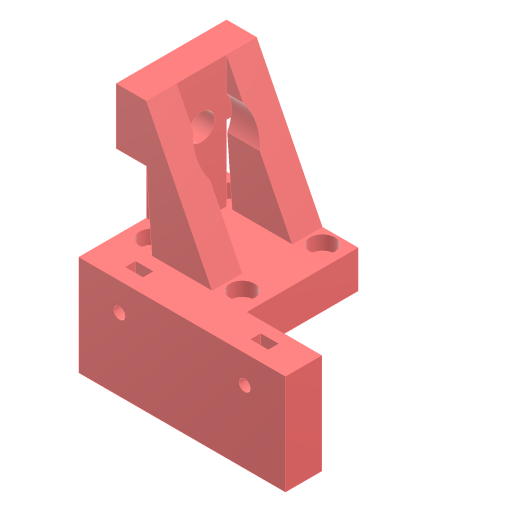
# Autodesk Inventor part: Part1
Saved by Autodesk Inventor 2024.3 (Build 283343000, 343)
## iProperties
Created: 2025-03-29
Part Number: Part1
Material: PC/ABS Plastic
Document SubType Name: Modeling
Designer: MPA
Density: 1.1 g/cm^3
Appearance: Smooth - Red
Mass: 105.816 g
Surface Area: 229.328 cm^2
Volume: 96.196 cm^3
Author: MPA
## iProperties of the stored document Part1_3DPrint.ipt
Created: 2025-06-18
Part Number: Part1_3DPrint
Material: Generic
Document SubType Name: Modeling
Designer: MPA
Density: 1 g/cm^3
Appearance: Default
Author: MPA
Autodesk Inventor part; units mm, degrees
ref_plane "YZ Plane" through (0, 0, 0) normal (1, 0, 0) x (0, 1, 0)
ref_plane "XZ Plane" through (0, 0, 0) normal (0, 1, 0) x (-1, 0, 0)
ref_plane "XY Plane" through (0, 0, 0) normal (0, 0, 1) x (1, 0, 0)
sketch "Sketch1" plane through (0, 0, 0) normal (0, 1, 0) x (-1, 0, 0)
  line L0 (-26.25, 22) -> (26.25, 22)
  line L1 (26.25, 22) -> (26.25, -22)
  line L2 (26.25, -22) -> (-26.25, -22)
  line L3 (-26.25, -22) -> (-26.25, 22)
  line L4 (-26.25, 22) -> (26.25, -22) construction
  line L5 (26.25, 22) -> (-26.25, -22) construction
  point P0 (0, 0)
  dimension "d0" = 44
  dimension "d1" = 52.5
  constraints: 12 end point, 2 midpoint, 2 parallel, 1 horizontal, 1 perpendicular
  measures "d0" distance of L0.end L1.end
  measures "d1" distance of L1.end L2.end
extrude "Extrusion1" add sketch "Sketch1" along normal blind 67.5
sketch "Sketch2" plane through (0, 67.5, 0) normal (0, 1, 0) x (1, 0, 0)
  line L0 (18, -16) -> (-18, -16) construction
  line L1 (-18, -16) -> (-18, 16) construction
  line L2 (-18, 16) -> (18, 16) construction
  line L3 (18, 16) -> (18, -16) construction
  line L4 (18, -16) -> (-18, 16) construction
  line L5 (-18, -16) -> (18, 16) construction
  point P0 (0, 0)
  point P1 (-18, 16)
  dimension "d4" = 32
  dimension "d5" = 36
  constraints: 12 end point, 4 coincident, 2 midpoint, 2 parallel, 1 horizontal, 1 perpendicular
  measures "d4" distance of L0.end L1.end
  measures "d5" distance of L1.end L2.end
hole "Hole1" at (-18, 67.5, -16) at (-18, 67.5, 16) at (18, 67.5, 16) at (18, 67.5, -16) direction (0, -1, 0) diameter 5.6 end through all
sketch "Sketch3" plane through (-26.25, 0, -22) normal (-1, 0, 0) x (0, 0, 1)
  line L0 (0, 0) -> (44, 0) projected
  line L1 (44, 0) -> (44, 67.5) projected
  line L2 (0, 67.5) -> (44, 67.5) projected
  line L3 (0, 0) -> (0, 67.5) projected
  point P0 (22, 0)
  point P1 (22, 47.5)
  point P2 (22, 0)
  dimension "d13" = 47.5
  constraints: 1 midpoint, 1 vertical alignment
  measures "d13" distance from line of L0 point (22, 47.5)
hole "Hole2" at (-26.25, 47.5, 0) direction (1, 0, 0) diameter 10.5 end through all
sketch "Sketch4" plane through (0, 67.5, 0) normal (0, 1, 0) x (1, 0, 0)
  circle A0 centre (18, 16) radius 2.8 projected
  circle A1 centre (18, -16) radius 2.8 projected
  circle A2 centre (-18, -16) radius 2.8 projected
  circle A3 centre (-18, 16) radius 2.8 projected
  line L0 (26.25, 22) -> (-26.25, 22) projected
  line L1 (-26.25, 22) -> (-26.25, -22) projected
  line L2 (-26.25, -22) -> (26.25, -22) projected
  line L3 (26.25, -22) -> (26.25, 22) projected
  line L4 (26.25, 22) -> (-14.25, 22)
  line L5 (-14.25, 22) -> (-14.25, -22)
  line L6 (-14.25, -22) -> (26.25, -22)
  line L7 (26.25, -22) -> (26.25, 22)
  line L8 (-26.25, 22) -> (-14.25, 22)
  line L9 (-14.25, 22) -> (-14.25, 10)
  line L10 (-14.25, 10) -> (-26.25, 10)
  line L11 (-26.25, 10) -> (-26.25, 22)
  line L12 (-14.25, -22) -> (-26.25, -22)
  line L13 (-26.25, -22) -> (-26.25, -10)
  line L14 (-26.25, -10) -> (-14.25, -10)
  line L15 (-14.25, -10) -> (-14.25, -22)
  point P0 (0, 0)
  dimension "d21" = 12
  dimension "d22" = 6
  dimension "d23" = 6
  dimension "d24" = 6
  constraints: 24 end point, 6 parallel, 3 horizontal, 3 perpendicular, 3 point on line
  measures "d21" distance between parallel lines of L1 L5
  measures "d22" distance from line of L0 A3.centre
  measures "d23" distance from line of L10 A3.centre
  measures "d24" distance from line of A2.centre L14
extrude "Extrusion2" cut sketch "Sketch4" against normal blind 52.5 contours L3 L2 L5 L0 | L5 L10 L1 L0 | L2 L1 L14 L5
sketch "Sketch5" plane through (-26.25, 67.5, 10) normal (0, 0, 1) x (1, 0, 0)
  line L0 (0, 0) -> (12, 0) projected
  line L1 (0, -52.5) -> (0, 0) projected
  line L2 (0, -52.5) -> (12, -52.5) projected
  line L3 (12, 0) -> (12, -52.5) projected
  line L4 (52.5, -52.5) -> (0, -52.5) projected
  line L5 (11.05, -52.5) -> (5.45, -52.5) projected
  line L6 (8.25, -52.5) -> (8.25, 0) construction
  line L7 (12, -22.5) -> (14.25, -52.5)
  line L8 (12, 0) -> (38.25, -52.5)
  line L9 (47.05, -52.5) -> (41.45, -52.5) projected
  line L10 (44.25, -52.5) -> (44.25, -22.1018) construction
  line L11 (12, -22.5) -> (0, -22.5)
  line L12 (0, -22.5) -> (0, 0)
  line L13 (0, 0) -> (12, 0)
  line L14 (38.25, -52.5) -> (14.25, -52.5)
  point P0 (26.25, -67.5)
  dimension "d27" = 30
  dimension "d28" = 36
  dimension "d29" = 6
  dimension "d30" = 6
  constraints: 16 end point, 5 point on line, 4 perpendicular, 2 midpoint, 1 collinear, 1 vertical
  measures "d27" distance from line of L4 L7.start
  measures "d28" distance between parallel lines of L10 L6
  measures "d29" distance from line of L10 L8.end
  measures "d30" distance from line of L6 L7.end
extrude "Extrusion3" add sketch "Sketch5" along normal up to surface (12 mm away) contours L0 L3 L11 L1 | L8 L4 L7 L3
sketch "Sketch6" plane through (0, 15, 0) normal (0, 1, 0) x (1, 0, 0)
  circle A0 centre (-18, -16) radius 2.8 projected
  circle A1 centre (18, -16) radius 2.8 projected
  circle A2 centre (18, 16) radius 2.8 projected
  circle A3 centre (-18, 16) radius 2.8 projected
  circle A4 centre (-18, 16) radius 2.8 projected
  point P0 (0, 0)
hole "Hole3" at (-18, 15, 16) at (18, 15, -16) at (-18, 15, -16) at (18, 15, 16) direction (0, -1, 0) diameter 5.5 end through all counterbore diameter 10 counterbore depth 5.7 clearance for "Socket Head Cap Screw ISO 4762" size "M5" standard "ISO"
mirror "Mirror1" about plane through (0, 0, 0) normal (0, 0, 1) of "Extrusion3"
sketch "Sketch7" plane through (-14.25, 15, 10) normal (1, 0, 0) x (0, 0, -1)
  circle A0 centre (10, 32.5) radius 5.25 projected
  circle A1 centre (10, 32.5) radius 12
  point P0 (10, -15)
  dimension "d40" = 24
  constraints: 1 centre point, 1 coincident
  measures "d40" diameter of A1
extrude "Extrusion4" cut sketch "Sketch7" along normal through all contours A0 | A1
sketch "Sketch8" plane through (-26.25, 0, 22) normal (0, 0, 1) x (1, 0, 0)
  line L0 (52.5, 15) -> (38.25, 15) projected
  line L1 (12, 67.5) -> (38.25, 15) projected
  line L2 (0, 67.5) -> (12, 67.5) projected
  line L3 (0, 45) -> (0, 67.5) projected
  line L4 (12, 45) -> (0, 45) projected
  line L5 (14.25, 15) -> (12, 45) projected
  line L6 (14.25, 15) -> (0, 15) projected
  line L7 (0, 0) -> (0, 15) projected
  line L8 (0, 0) -> (52.5, 0) projected
  line L9 (52.5, 0) -> (52.5, 15) projected
  line L10 (14.25, 15) -> (38.25, 15)
  point P0 (26.25, 0)
  constraints: 2 end point, 1 collinear
extrude "Extrusion5" add sketch "Sketch8" along normal blind 15 contours L9 L8 L7 L6 L10 L0
sketch "Sketch9" plane through (0, 0, 0) normal (0, -1, 0) x (1, 0, 0)
  circle A0 centre (18, -16) radius 2.8 projected
  circle A1 centre (18, 16) radius 2.8 projected
  circle A2 centre (-18, 16) radius 2.8 projected
  circle A3 centre (-18, -16) radius 2.8 projected
  line L0 (26.25, -22) -> (-26.25, -22) projected
  line L1 (26.25, -22) -> (26.25, 37) projected
  line L2 (-26.25, 37) -> (26.25, 37) projected
  line L3 (-26.25, -22) -> (-26.25, 37) projected
  line L4 (-26.25, 22.5) -> (27.0192, 22.5)
  point P0 (0, 0)
  point P1 (26.25, 22.5)
  dimension "d45" = 14.5
  constraints: 2 end point, 1 perpendicular, 1 point on line
  measures "d45" distance between parallel lines of L2 L4
extrude "Extrusion6" add sketch "Sketch9" along normal blind 25 contours L4 L3 L2 L1
sketch "Sketch10" plane through (26.25, 0, -22) normal (1, 0, 0) x (0, 0, -1)
  line L0 (0, 15) -> (-59, 15) projected
  line L1 (-59, 15) -> (-59, -25) projected
  line L2 (-44.5, -25) -> (-59, -25) projected
  line L3 (-44.5, 0) -> (-44.5, -25) projected
  line L4 (0, 0) -> (-44.5, 0) projected
  line L5 (0, 0) -> (0, 15) projected
  line L6 (-44.5, 0) -> (-44.5, 15)
  point P0 (-22, 0)
  constraints: 2 end point, 1 perpendicular, 1 point on line
extrude "Extrusion7" add sketch "Sketch10" along normal blind 30 contours L6 L3 L2 L1 L0
sketch "Sketch11" plane through (-26.25, 0, 37) normal (0, 0, 1) x (1, 0, 0)
  line L0 (0, 15) -> (0, -25) projected
  line L1 (0, -25) -> (82.5, -25) projected
  line L2 (82.5, 15) -> (82.5, -25) projected
  line L3 (0, 15) -> (82.5, 15) projected
  line L4 (0, 15) -> (82.5, -25) construction
  line L5 (82.5, 15) -> (0, -25) construction
  line L6 (-31.1297, -30) -> (116.2871, -30) construction
  point P0 (26.25, 0)
  point P1 (16.25, 3.8)
  point P2 (66.25, 3.8)
  point P3 (41.25, -5)
  dimension "d50" = 50
  dimension "d51" = 25
  dimension "d52" = 5
  dimension "d53" = 33.8
  constraints: 6 end point, 1 horizontal, 1 horizontal alignment, 1 midpoint
  measures "d50" distance of point (66.25, 3.8) point (16.25, 3.8)
  measures "d51" horizontal distance of point (41.25, -5) point (16.25, 3.8)
  measures "d52" distance between parallel lines of L1 L6
  measures "d53" distance from line of L6 point (16.25, 3.8)
hole "Hole4" at (-10, 3.8, 37) at (40, 3.8, 37) direction (0, 0, -1) diameter 4.6 depth 10
sketch "Sketch12" plane through (40, 3.8, 27) normal (0, 0, 1) x (1, 0, 0)
  circle A0 centre (0, 0) radius 2.3 projected
  circle A1 centre (-50, 0) radius 2.3 projected
  line L0 (-46.4, 2.0785) -> (-46.4, -2.0785)
  line L1 (-46.4, -2.0785) -> (-50, -4.1569)
  line L2 (-50, -4.1569) -> (-53.6, -2.0785)
  line L3 (-53.6, -2.0785) -> (-53.6, 2.0785)
  line L4 (-53.6, 2.0785) -> (-50, 4.1569)
  line L5 (-50, 4.1569) -> (-46.4, 2.0785)
  line L6 (0, 4.1569) -> (3.6, 2.0785)
  line L7 (3.6, 2.0785) -> (3.6, -2.0785)
  line L8 (3.6, -2.0785) -> (0, -4.1569)
  line L9 (0, -4.1569) -> (-3.6, -2.0785)
  line L10 (-3.6, -2.0785) -> (-3.6, 2.0785)
  line L11 (-3.6, 2.0785) -> (0, 4.1569)
  line L12 (-66.25, 11.2) -> (16.25, 11.2) projected
  line L13 (-53.6, 2.0785) -> (-53.6, 11.2)
  line L14 (-46.4, 2.0785) -> (-46.4, 11.2)
  line L15 (-3.6, 2.0785) -> (-3.6, 11.2)
  line L16 (3.6, 2.0785) -> (3.6, 11.2)
  point P0 (-40, -3.8)
  point P1 (-50, 0)
  dimension "d61" = 7.2
  constraints: 32 end point, 4 perpendicular, 4 point on line, 2 coincident, 2 vertical alignment, 1 parallel, 26 other
  measures "d61" distance between parallel lines of L0 L3
extrude "Extrusion8" cut sketch "Sketch12" along normal blind 4.2
sketch "Sketch13" plane through (-13.6, 1.7215, 27) normal (0, 0, 1) x (1, 0, 0)
  circle A0 centre (3.6, 2.0785) radius 2.3 projected
  circle A1 centre (3.6, 2.0785) radius 2.3 projected
  circle A2 centre (53.6, 2.0785) radius 2.3 projected
  circle A3 centre (53.6, 2.0785) radius 2.3 projected
  point P0 (13.6, -1.7215)
hole "Hole5" at (-10, 3.8, 27) at (40, 3.8, 27) direction (0, 0, -1) diameter 4.6 depth 5
equation "\"d23\" = d22"
equation "\"d24\" = d23"
equation "\"d30\" = d29"
equation "\"d51\" = 0.5 * d50"
body "Solid1"
